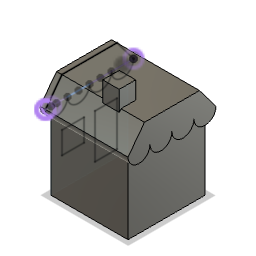
MMEZP_Obchudek v4 (Autodesk Fusion 360 design; units mm, degrees)
Autodesk Fusion 360 part; units mm, degrees
note: some values were not read from the file. Set by a fixed rule: which sketch regions a step uses.
sketch "Sketch1" plane through (0, 0, 0) normal (0, 1, 0) x (1, 0, 0)
  line L0 (0, 0) -> (35, 0)
  line L1 (35, 0) -> (35, -35)
  line L2 (35, -35) -> (0, -35)
  line L3 (0, -35) -> (0, 0)
  line L4 (3.2, -3.2) -> (31.8, -3.2)
  line L5 (31.8, -3.2) -> (31.8, -31.8)
  line L6 (31.8, -31.8) -> (3.2, -31.8)
  line L7 (3.2, -31.8) -> (3.2, -3.2)
  dimension "d1" = 35
  dimension "d2" = 3.2
  dimension "d3" = 3.2
  dimension "d4" = 35
  dimension "d5" = 3.2
  dimension "d6" = 3.2
  constraint horizontal L0
  constraint vertical L1
  constraint horizontal L2
  constraint vertical L3
  constraint coincident L0.start L3.end
  constraint horizontal L4
  constraint vertical L5
  constraint horizontal L6
  constraint vertical L7
  measures "d1" distance of L0.start L0.end
  measures "d2" distance of L0 L4
  measures "d3" distance of L3 L7
  measures "d4" distance of L0.start L2.end
  measures "d5" distance of L2 L6
  measures "d6" distance of L1 L5
extrude "Extrude1" add sketch "Sketch1" along normal blind 35 makes body 1
sketch "Sketch2" plane through (0, 35, 0) normal (0, 1, 0) x (-1, 0, 0)
  line L0 (-31.8, 31.8) -> (-3.2, 31.8)
  line L1 (-3.2, 31.8) -> (-3.2, 3.2)
  line L2 (-3.2, 3.2) -> (-31.8, 3.2)
  line L3 (-31.8, 3.2) -> (-31.8, 31.8)
  line L4 (0, 35) -> (-35, 35)
  line L5 (-35, 35) -> (-35, 0)
  line L6 (-35, 0) -> (0, 0)
  line L7 (0, 0) -> (0, 35)
  line L8 (2.5, -2.5) -> (-37.5, -2.5)
  line L9 (-37.5, -2.5) -> (-37.5, 37.5)
  line L10 (-37.5, 37.5) -> (2.5, 37.5)
  line L11 (2.5, 37.5) -> (2.5, -2.5)
  line L12 (-26.8, 30.8) -> (-19.3, 30.8)
  line L13 (-19.3, 30.8) -> (-19.3, 23.3)
  line L14 (-19.3, 23.3) -> (-26.8, 23.3)
  line L15 (-26.8, 23.3) -> (-26.8, 30.8)
  line L16 (-31.8, 31.8) -> (-3.2, 31.8)
  line L17 (-31.8, 3.2) -> (-31.8, 31.8)
  dimension "d9" = 2.5
  dimension "d10" = 2.5
  dimension "d11" = 2.5
  dimension "d12" = 2.5
  dimension "d54" = 7.5
  dimension "d55" = 7.5
  dimension "d56" = 1
  dimension "d57" = 5
  constraint horizontal L8
  constraint vertical L9
  constraint horizontal L10
  constraint vertical L11
  constraint horizontal L12
  constraint vertical L13
  constraint horizontal L14
  constraint vertical L15
  measures "d9" distance of L6 L8
  measures "d10" distance of L7 L11
  measures "d11" distance of L4 L10
  measures "d12" distance of L5 L9
  measures "d54" distance of L12.start L12.end
  measures "d55" distance of L12.end L13.end
  measures "d56" distance of L12 L16
  measures "d57" distance of L15 L17
sketch "Sketch3" plane through (0, 35, 0) normal (0, 1, 0) x (-1, 0, 0)
sketch "Sketch4" plane through (0, 0, 0) normal (-1, 0, 0) x (0, 0, 1)
  line L0 (0, 0) -> (35, 0)
  line L1 (35, 0) -> (35, 35)
  line L2 (35, 35) -> (0, 35)
  line L3 (0, 35) -> (0, 0)
  line L4 (-2.5, 35) -> (7.5, 35)
  arc A0 (-2.5, 35) -> (7.5, 35) centre (2.5, 35.0004) ccw
  arc A1 (7.5, 35) -> (17.5, 35) centre (12.5, 35) ccw
  arc A2 (17.5, 35) -> (27.5, 35) centre (22.5, 35) ccw
  line L5 (27.5, 35) -> (27.5, 35)
  line L6 (-2.5, 35) -> (5, 45)
  line L7 (5, 45) -> (30, 45)
  line L8 (5, 23.2) -> (15, 23.2)
  line L9 (15, 23.2) -> (15, 3.2)
  line L10 (15, 3.2) -> (5, 3.2)
  line L11 (5, 3.2) -> (5, 23.2)
  line L12 (20, 23.2) -> (30, 23.2)
  line L13 (30, 23.2) -> (30, 13.2)
  line L14 (30, 13.2) -> (20, 13.2)
  line L15 (20, 13.2) -> (20, 23.2)
  line L16 (7.5, 35) -> (17.5, 35)
  line L17 (27.5, 35) -> (17.5, 35)
  line L18 (35, 35) -> (37.5, 35)
  arc A3 (27.5, 35) -> (37.5, 35) centre (32.5, 35) ccw
  line L19 (37.5, 35) -> (30, 45)
  line L20 (37.5, 35) -> (-2.5, 35)
  point P0 (35, 35)
  point P1 (37.5, 35)
  dimension "d13" = 10
  dimension "d14" = 5
  dimension "d15" = 10
  dimension "d16" = 10
  dimension "d18" = 7.5
  dimension "d22" = 10
  dimension "d23" = 20
  dimension "d24" = 3.2
  dimension "d25" = 5
  dimension "d26" = 5
  dimension "d27" = 10
  dimension "d28" = 10
  dimension "d29" = 13.2
  dimension "d31" = 10
  dimension "d33" = 7.5
  dimension "d35" = 40
  dimension "d36" = 10
  constraint coincident L4.start A0.start
  constraint coincident L2 L4.end
  constraint coincident L2 A1.centre
  constraint coincident L2 A1.end
  constraint coincident L2 A2.centre
  constraint coincident L2 A2.end
  constraint parallel L4 L7
  constraint horizontal L8
  constraint vertical L9
  constraint horizontal L10
  constraint vertical L11
  constraint horizontal L12
  constraint vertical L13
  constraint horizontal L14
  constraint vertical L15
  constraint coincident L2 A3.centre
  constraint coincident P0 L1.end
  constraint perpendicular L1 L18
  measures "d13" diameter of A0
  measures "d14" horizontal distance of A0.centre L4.start
  measures "d15" diameter of A1
  measures "d16" diameter of A2
  measures "d18" horizontal distance of L4.start L6.end
  measures "d22" distance of L8.start L8.end
  measures "d23" distance of L8.start L10.end
  measures "d24" distance of L0 L10
  measures "d25" distance of L3 L11
  measures "d26" distance of L1 L13
  measures "d27" distance of L12 L14
  measures "d28" distance of L13 L15
  measures "d29" distance of L0 L14
  measures "d31" diameter of A3
  measures "d33" horizontal distance of L7.end P1
  measures "d35" distance of L4.start P1
  measures "d36" distance of L7 L20
extrude "Extrude2" add sketch "Sketch1" along normal blind 3.2 contours L4 L5 L6 L7 bodies 1
extrude "Extrude3" cut sketch "Sketch4" against normal blind 3.2 contours L8 L9 L10 L11 bodies 1
extrude "Extrude4" cut sketch "Sketch4" against normal blind 3.2 contours L12 L13 L14 L15 bodies 1
extrude "Extrude5" add sketch "Sketch4" along normal blind 2.5 separate body contours L3 L4 A0 L20 | L2 L3 L4 A0 L20 | L1 L2 A3 L20 | L1 L18 A3 L20 | L2 L4 L6 L7 L16 L17 L18 L19 L20 | L2 A1 L16 L20 | L2 A2 L17 L20 makes body 2
extrude "Extrude6" add sketch "Sketch4" against normal blind 37.5 contours L3 L4 A0 L20 bodies 1 2
extrude "Extrude7" add sketch "Sketch4" against normal blind 37.5 separate body contours L1 L18 A3 L20 makes body 3
extrude "Extrude8" add sketch "Sketch4" against normal blind 37.5 contours L2 L4 L6 L7 L16 L17 L18 L19 L20 bodies 1 3
extrude "Extrude9" add sketch "Sketch4" against normal blind 2.5 from surface at -35 contours L2 L3 L4 A0 L20 | L1 L2 A3 L20 | L2 A1 L16 L20 | L2 A2 L17 L20 bodies 1
extrude "Extrude10" add sketch "Sketch2" along normal blind 18 contours L12 L13 L14 L15 bodies 1
